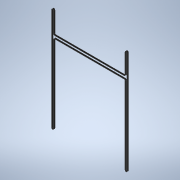
# Autodesk Inventor part: gt2_belt
Saved by Autodesk Inventor 2021 (Build 250183000, 183)
## iProperties
Created: 2023-01-31
Part Number: gt2_belt
Material: Типовые
Document SubType Name: Modeling
Designer: ignat
Density: 1 g/cm^3
Appearance: По умолчанию
Author: ignat
Autodesk Inventor part; units mm, degrees
ref_plane "YZ Plane" through (0, 0, 0) normal (1, 0, 0) x (0, 1, 0)
ref_plane "XZ Plane" through (0, 0, 0) normal (0, 1, 0) x (-1, 0, 0)
ref_plane "XY Plane" through (0, 0, 0) normal (0, 0, 1) x (1, 0, 0)
sketch "Эскиз1" plane through (0, 0, 0) normal (0, 0, 1) x (1, 0, 0)
  arc A0 (68.75, 375.75) -> (58.75, 375.75) centre (63.75, 375.75) ccw
  arc A1 (53.75, 266.5202) -> (58.75, 271.5202) centre (53.75, 271.5202) ccw
  arc A2 (58.75, 246.5202) -> (53.75, 251.5202) centre (53.75, 246.5202) ccw
  arc A3 (-312.25, 375.75) -> (-322.25, 375.75) centre (-317.25, 375.75) ccw
  arc A4 (-312.25, 271.5202) -> (-307.25, 266.5202) centre (-307.25, 271.5202) ccw
  arc A5 (-307.25, 251.5202) -> (-312.25, 246.5202) centre (-307.25, 246.5202) ccw
  arc A6 (-322.25, -155.2817) -> (-312.25, -155.2817) centre (-317.25, -155.2817) ccw
  arc A7 (58.75, -155.2817) -> (68.75, -155.2817) centre (63.75, -155.2817) ccw
  line L0 (68.75, -155.2817) -> (68.75, 375.75)
  line L1 (58.75, 375.75) -> (58.75, 271.5202)
  line L2 (53.75, 266.5202) -> (-307.25, 266.5202)
  line L3 (-307.25, 251.5202) -> (53.75, 251.5202)
  line L4 (58.75, 246.5202) -> (58.75, -155.2817)
  line L5 (-312.25, -155.2817) -> (-312.25, 246.5202)
  line L6 (-312.25, 271.5202) -> (-312.25, 375.75)
  line L7 (-322.25, 375.75) -> (-322.25, -155.2817)
  line L8 (-307.25, 267.0202) -> (53.75, 267.0202)
  arc A8 (53.75, 267.0202) -> (58.25, 271.5202) centre (53.75, 271.5202) ccw
  line L9 (58.25, 271.5202) -> (58.25, 375.75)
  arc A9 (69.25, 375.75) -> (58.25, 375.75) centre (63.75, 375.75) ccw
  line L10 (69.25, 375.75) -> (69.25, -155.2817)
  arc A10 (58.25, -155.2817) -> (69.25, -155.2817) centre (63.75, -155.2817) ccw
  line L11 (58.25, -155.2817) -> (58.25, 246.5202)
  arc A11 (58.25, 246.5202) -> (53.75, 251.0202) centre (53.75, 246.5202) ccw
  line L12 (53.75, 251.0202) -> (-307.25, 251.0202)
  arc A12 (-307.25, 251.0202) -> (-311.75, 246.5202) centre (-307.25, 246.5202) ccw
  line L13 (-311.75, 246.5202) -> (-311.75, -155.2817)
  arc A13 (-322.75, -155.2817) -> (-311.75, -155.2817) centre (-317.25, -155.2817) ccw
  line L14 (-322.75, -155.2817) -> (-322.75, 375.75)
  arc A14 (-311.75, 375.75) -> (-322.75, 375.75) centre (-317.25, 375.75) ccw
  line L15 (-311.75, 375.75) -> (-311.75, 271.5202)
  arc A15 (-311.75, 271.5202) -> (-307.25, 267.0202) centre (-307.25, 271.5202) ccw
  line L16 (-307.25, 266.0202) -> (53.75, 266.0202)
  arc A16 (53.75, 266.0202) -> (59.25, 271.5202) centre (53.75, 271.5202) ccw
  line L17 (59.25, 271.5202) -> (59.25, 375.75)
  arc A17 (68.25, 375.75) -> (59.25, 375.75) centre (63.75, 375.75) ccw
  line L18 (68.25, 375.75) -> (68.25, -155.2817)
  arc A18 (59.25, -155.2817) -> (68.25, -155.2817) centre (63.75, -155.2817) ccw
  line L19 (59.25, -155.2817) -> (59.25, 246.5202)
  arc A19 (59.25, 246.5202) -> (53.75, 252.0202) centre (53.75, 246.5202) ccw
  line L20 (53.75, 252.0202) -> (-307.25, 252.0202)
  arc A20 (-307.25, 252.0202) -> (-312.75, 246.5202) centre (-307.25, 246.5202) ccw
  line L21 (-312.75, 246.5202) -> (-312.75, -155.2817)
  arc A21 (-321.75, -155.2817) -> (-312.75, -155.2817) centre (-317.25, -155.2817) ccw
  line L22 (-321.75, -155.2817) -> (-321.75, 375.75)
  arc A22 (-312.75, 375.75) -> (-321.75, 375.75) centre (-317.25, 375.75) ccw
  line L23 (-312.75, 375.75) -> (-312.75, 271.5202)
  arc A23 (-312.75, 271.5202) -> (-307.25, 266.0202) centre (-307.25, 271.5202) ccw
  point P0 (70, 190)
  dimension "d0" = 0.5
  dimension "d1" = 0.5
  constraints: 48 end point, 48 point on circle, 24 centre point, 4 point on line
  measures "d0" distance between parallel lines of L2 L8
  measures "d1" distance between parallel lines of L2 L16
extrude "Выдавливание1" add sketch "Эскиз1" along normal blind 7 contours L0 A7 L4 A2 L3 A5 L5 A6 L7 A3 L6 A4 L2 A1 L1 A0 | L8 A8 L9 A9 L10 A10 L11 A11 L12 A12 L13 A13 L14 A14 L15 A15
